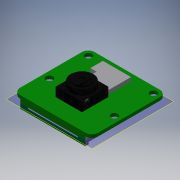
# Autodesk Inventor part: Raspberry Camera V2.1
Saved by Autodesk Inventor 2017 (Build 210142000, 142)
## iProperties
Part Number: Raspberry Camera V2.1
Material: Generisch
Document SubType Name: Modeling
Designer: David Merges
Density: 1 g/cm^3
Appearance: Vorgabe
Author: David Merges
Autodesk Inventor part; units mm, degrees
ref_plane "YZ Plane" through (0, 0, 0) normal (1, 0, 0) x (0, 1, 0)
ref_plane "XZ Plane" through (0, 0, 0) normal (0, 1, 0) x (-1, 0, 0)
ref_plane "XY Plane" through (0, 0, 0) normal (0, 0, 1) x (1, 0, 0)
sketch "Skizze1" plane through (0, 0, 0) normal (0, 0, 1) x (1, 0, 0)
  line L0 (-10.5, 14.5) -> (10.5, 14.5)
  line L1 (12.5, 12.5) -> (12.5, -7.362)
  line L2 (10.5, -9.362) -> (-10.5, -9.362)
  line L3 (-12.5, -7.362) -> (-12.5, 12.5)
  line L4 (-10.4, 12.5) -> (10.4, 12.5) construction
  line L5 (10.4, 12.5) -> (10.4, 0) construction
  line L6 (10.4, 0) -> (-10.4, 0) construction
  line L7 (-10.4, 0) -> (-10.4, 12.5) construction
  circle A0 centre (-10.4, 12.5) radius 1.1
  circle A1 centre (10.4, 12.5) radius 1.1
  circle A2 centre (-10.4, 0) radius 1.1
  circle A3 centre (10.4, 0) radius 1.1
  arc A4 (-10.5, 14.5) -> (-12.5, 12.5) centre (-10.5, 12.5) ccw
  arc A5 (12.5, 12.5) -> (10.5, 14.5) centre (10.5, 12.5) ccw
  arc A6 (10.5, -9.362) -> (12.5, -7.362) centre (10.5, -7.362) ccw
  arc A7 (-12.5, -7.362) -> (-10.5, -9.362) centre (-10.5, -7.362) ccw
  line L8 (0, -9.362) -> (0, 0) construction
  point P0 (-12.5, 14.5)
  point P1 (12.5, -9.362)
  point P2 (-12.5, -9.362)
  dimension "d0" = 25
  dimension "d1" = 23.862
  dimension "d2" = 2.2
  dimension "d3" = 2
  dimension "d4" = 20.8
  dimension "d5" = 12.5
  dimension "d6" = 2
  constraints: 18 end point, 8 centre point, 8 point on circle, 8 tangent, 6 equal radius, 6 point on line, 5 coincident, 4 parallel, 3 perpendicular, 2 horizontal, 2 midpoint
  measures "d0" distance of point (12.5, -9.362) point (-12.5, -9.362)
  measures "d1" distance of point (-12.5, -9.362) point (-12.5, 14.5)
  measures "d2" diameter of A0
  measures "d3" radius of A4
  measures "d4" distance between parallel lines of L5 L7
  measures "d5" distance of L4.end L5.end
  measures "d6" distance between parallel lines of L0 L4
extrude "Extrusion1" add sketch "Skizze1" along normal mid plane 1
sketch "Skizze2" plane through (0, 0, 0.5) normal (0, 0, 1) x (1, 0, 0)
  line L0 (-4.2, 4.2) -> (4.2, 4.2)
  line L1 (4.2, 4.2) -> (4.2, -4.2)
  line L2 (4.2, -4.2) -> (-4.2, -4.2)
  line L3 (-4.2, -4.2) -> (-4.2, 4.2)
  line L4 (-4.2, -4.2) -> (4.2, 4.2) construction
  point P0 (0, 0)
  point P1 (0, 0)
  dimension "d9" = 8.4
  constraints: 10 end point, 2 parallel, 2 perpendicular, 1 coincident, 1 horizontal, 1 midpoint
  measures "d9" distance of L1.end L2.end
extrude "Extrusion2" add sketch "Skizze2" along normal blind 2.9
sketch "Skizze3" plane through (0, 0, 3.4) normal (0, 0, 1) x (1, 0, 0)
  circle A0 centre (0, 0) radius 3.6
  dimension "d12" = 7.2
  constraints: 1 centre point, 1 coincident
  measures "d12" diameter of A0
extrude "Extrusion3" add sketch "Skizze3" along normal blind 1.7
sketch "Skizze4" plane through (0, 0, 5.1) normal (0, 0, 1) x (1, 0, 0)
  circle A0 centre (0, 0) radius 2.7
  circle A1 centre (0, 0) radius 0.85
  dimension "d15" = 5.4
  dimension "d16" = 1.7
  constraints: 2 centre point, 2 coincident
  measures "d15" diameter of A0
  measures "d16" diameter of A1
extrude "Extrusion4" add sketch "Skizze4" along normal blind 0.5
sketch "Skizze5" plane through (0, 0, 0.5) normal (0, 0, 1) x (1, 0, 0)
  point P0 (0, 0)
sketch "Skizze6" plane through (0, 0, 0.5) normal (0, 0, 1) x (1, 0, 0)
  line L0 (4.2, 4.2) -> (-4.2, 4.2) projected
  line L1 (-3.5, 4.2) -> (3.5, 4.2)
  line L2 (3.5, 4.2) -> (3.5, 12.2)
  line L3 (3.5, 12.2) -> (-2.9111, 12.2)
  line L4 (-2.9111, 12.2) -> (-5.5, 12.2)
  line L5 (-5.5, 12.2) -> (-5.5, 8.2)
  line L6 (-5.5, 8.2) -> (-3.5, 8.2)
  line L7 (-3.5, 8.2) -> (-3.5, 4.2)
  point P0 (0, 0)
  point P1 (0, 4.2)
  dimension "d19" = 9
  dimension "d20" = 7
  dimension "d21" = 4
  dimension "d22" = 8
  constraints: 14 end point, 3 parallel, 2 horizontal, 2 midpoint, 2 perpendicular, 1 point on line
  measures "d19" distance between parallel lines of L5 L2
  measures "d20" distance between parallel lines of L2 L7
  measures "d21" distance of L4.end L5.end
  measures "d22" distance between parallel lines of L3 L0
extrude "Extrusion5" add sketch "Skizze6" along normal blind 1.2
sketch "Skizze7" plane through (0, 0, -0.5) normal (0, 0, -1) x (-1, 0, 0)
  line L0 (-10.5, -9.362) -> (10.5, -9.362) projected
  line L1 (10.5, -9.362) -> (-10.5, -9.362) projected
  line L2 (10.4, -9.362) -> (-10.4, -9.362)
  line L3 (-10.4, -9.362) -> (-10.4, -8.212)
  line L4 (-10.4, -8.212) -> (10.4, -8.212)
  line L5 (10.4, -8.212) -> (10.4, -9.362)
  line L6 (9.75, -8.212) -> (-9.75, -8.212)
  line L7 (-9.75, -8.212) -> (-9.75, -3.762)
  line L8 (-9.75, -3.762) -> (9.75, -3.762)
  line L9 (9.75, -3.762) -> (9.75, -8.212)
  point P0 (0, 0)
  point P1 (0, -9.362)
  point P2 (0, -8.212)
  dimension "d25" = 20.8
  dimension "d26" = 1.15
  dimension "d27" = 19.5
  dimension "d28" = 5.6
  constraints: 16 end point, 4 midpoint, 4 parallel, 2 horizontal, 2 perpendicular, 2 point on line
  measures "d25" distance between parallel lines of L3 L5
  measures "d26" distance between parallel lines of L0 L4
  measures "d27" distance between parallel lines of L9 L7
  measures "d28" distance between parallel lines of L0 L8
extrude "Extrusion6" add sketch "Skizze7" along normal blind 2.75
sketch "Skizze8" plane through (-10.5, -9.362, 0.5) normal (0, -1, 0) x (1, 0, 0)
  line L0 (21, 0) -> (21, -1) projected
  line L1 (0, 0) -> (21, 0) projected
  line L2 (0, 0) -> (0, -1) projected
  line L3 (0.1, -1) -> (0, -1) projected
  line L4 (0.1, -1) -> (0.1, -3.75) projected
  line L5 (20.9, -3.75) -> (0.1, -3.75) projected
  line L6 (20.9, -1) -> (20.9, -3.75) projected
  line L7 (21, -1) -> (20.9, -1) projected
  line L8 (2.5, -2.18) -> (18.5, -2.18)
  line L9 (18.5, -2.18) -> (18.5, -2.55)
  line L10 (18.5, -2.55) -> (2.5, -2.55)
  line L11 (2.5, -2.55) -> (2.5, -2.18)
  line L12 (0.75, -3.75) -> (20.25, -3.75) construction
  line L13 (10.5, -3.75) -> (10.5, -2.55) construction
  line L14 (20.9, -3.75) -> (0.1, -3.75) construction
  point P0 (10.5, -0.5)
  dimension "d31" = 1.2
  dimension "d32" = 0.37
  dimension "d33" = 16
  constraints: 10 end point, 2 midpoint, 2 parallel, 2 perpendicular, 1 horizontal
  measures "d31" distance between parallel lines of L10 L5
  measures "d32" distance between parallel lines of L8 L10
  measures "d33" distance of L8.start L8.end
extrude "Extrusion7" cut sketch "Skizze8" against normal blind 3.5 contours L8 L9 L10 L11
ref_plane "SMD component height" through (0, 0, -1.7) normal (0, 0, -1) x (-1, 0, 0)
sketch "Skizze10" plane through (0, 0, -0.5) normal (0, 0, -1) x (-1, 0, 0)
  line L0 (12.5079, -9.362) -> (-12.5079, -9.362) construction
  line L1 (-12.5079, -9.362) -> (-12.5079, 14.5) construction
  line L2 (-12.5079, 14.5) -> (12.5079, 14.5) construction
  line L3 (12.5079, 14.5) -> (12.5079, -9.362) construction
  line L4 (10.5, 14.5) -> (-10.5, 14.5) projected
  line L5 (-10.4, -9.362) -> (10.4, -9.362) projected
  point P0 (0, 0)
  point P1 (0, 14.5)
  point P2 (0, -9.362)
  constraints: 4 midpoint, 2 other
decal "Aufkleber1"
sketch "Skizze11" plane through (0, 0, -3.25) normal (0, 0, -1) x (-1, 0, 0)
  line L0 (10.5, 14.5) -> (-10.5, 14.5) projected
  line L1 (12.5079, -9.362) -> (-12.5079, -9.362) construction
  line L2 (-12.5079, -9.362) -> (-12.5079, 14.5) construction
  line L3 (-12.5079, 14.5) -> (12.5079, 14.5) construction
  line L4 (12.5079, 14.5) -> (12.5079, -9.362) construction
  line L5 (-10.4, -9.362) -> (10.4, -9.362) projected
  point P0 (0, 0)
  point P1 (0, -9.362)
  point P2 (0, 14.5)
  constraints: 4 midpoint, 2 other
decal "Aufkleber2"
sketch "Skizze12" plane through (-10.5, -9.362, 0.5) normal (0, -1, 0) x (1, 0, 0)
  line L0 (20.9, -1) -> (20.9, -3.75) projected
  line L1 (0.1, -1) -> (0.1, -3.75) projected
  line L2 (20.9, -1) -> (0.1, -1)
  line L3 (0.1, -1) -> (0.1, -1.01)
  line L4 (0.1, -1.01) -> (20.9, -1.01)
  line L5 (20.9, -1.01) -> (20.9, -1)
  point P0 (10.5, -0.5)
  dimension "d58" = 0.01
  constraints: 8 end point, 2 parallel, 1 horizontal, 1 perpendicular, 1 point on line
  measures "d58" distance between parallel lines of L4 L2
extrude "Extrusion9" cut sketch "Skizze12" against normal blind 0.01
